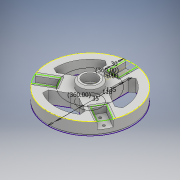
# Autodesk Inventor part: Base1
Saved by Autodesk Inventor 2017 (Build 210142000, 142)
## iProperties
Created: 2016-12-27
Part Number: Base1
Material: Generic
Document SubType Name: Modeling
Designer: Samanth
Density: 1 g/cm^3
Appearance: Default
Author: Samanth
Autodesk Inventor part; units mm, degrees
ref_plane "YZ Plane" through (0, 0, 0) normal (1, 0, 0) x (0, 1, 0)
ref_plane "XZ Plane" through (0, 0, 0) normal (0, 1, 0) x (-1, 0, 0)
ref_plane "XY Plane" through (0, 0, 0) normal (0, 0, 1) x (1, 0, 0)
sketch "Sketch1" plane through (0, 0, 0) normal (0, 0, 1) x (1, 0, 0)
  circle A0 centre (0, 0) radius 55
  circle A1 centre (0, 0) radius 17.5
  line L0 (-17.5, 0) -> (-17.5, 52.1416)
  line L1 (17.5, 0) -> (17.5, 52.1416)
  line L2 (8.75, -15.1554) -> (-36.406, -41.2263)
  line L3 (-8.75, 15.1554) -> (-53.906, -10.9154)
  circle A2 centre (0, 0) radius 17.5
  circle A3 centre (0, 0) radius 55
  line L4 (8.75, 15.1554) -> (53.906, -10.9154)
  line L5 (-8.75, -15.1554) -> (36.406, -41.2263)
  circle A4 centre (0, 0) radius 17.5
  circle A5 centre (0, 0) radius 55
  circle A6 centre (0, 0) radius 67.5
  line L6 (-36.406, -41.2263) -> (0, -20.2073)
  line L7 (36.406, -41.2263) -> (0, -20.2073)
  line L8 (53.906, -10.9154) -> (17.5, 10.1036)
  line L9 (17.5, 10.1036) -> (17.5, 52.1416)
  line L10 (-17.5, 10.1036) -> (-53.906, -10.9154)
  line L11 (-17.5, 52.1416) -> (-17.5, 10.1036)
  circle A7 centre (0, 0) radius 20.2073
  dimension "d0" = 110
  dimension "d1" = 35
  dimension "d4" = 360
  dimension "d6" = 135
  constraints: 24 end point, 12 point on circle, 8 coincident, 7 centre point, 6 point on line, 4 collinear, 2 tangent, 1 parallel, 1 vertical, 32 other
  measures "d0" diameter of A0
  measures "d1" diameter of A1
  measures "d6" diameter of A6
sketch "Sketch2" plane through (0, 0, 0) normal (0, 0, 1) x (1, 0, 0)
  circle A0 centre (0, 0) radius 67.5
  arc A1 (-17.5, 52.1416) -> (17.5, 52.1416) centre (0, 0) ccw
  line L0 (-17.5, 52.1416) -> (-17.5, 10.0984)
  line L1 (17.5, 10.0245) -> (17.5, 52.1416)
  line L2 (-36.406, -41.2263) -> (0, -20.2037)
  line L3 (-53.9044, -10.9232) -> (-17.5, 10.0984)
  arc A2 (-53.9044, -10.9232) -> (-36.406, -41.2263) centre (0, 0) ccw
  arc A3 (36.406, -41.2263) -> (53.906, -10.9154) centre (-0.0004, 0.0003) ccw
  arc A4 (-17.5, 52.1416) -> (17.5, 52.1416) centre (0, 0) ccw
  line L4 (36.406, -41.2263) -> (0, -20.2037)
  line L5 (-8.4334, -15.3339) -> (-9.065, -14.9691)
  line L6 (53.906, -10.9154) -> (17.5, 10.0245)
  arc A5 (-9.065, -14.9691) -> (-8.4334, -15.3339) centre (0, 0) ccw
  dimension "d7" = 135
  dimension "d8" = 110
  constraints: 14 end point, 13 point on circle, 6 centre point, 3 coincident, 2 parallel, 1 concentric
  measures "d7" diameter of A0
  measures "d8" diameter of A1
extrude "Extrusion1" add sketch "Sketch2" along normal blind 20 contours A0 | L6 L1 A1
sketch "Sketch3" plane through (0, 0, 20) normal (0, 0, 1) x (1, 0, 0)
  arc A0 (11.1455, 13.4917) -> (5.9543, 16.4559) centre (0, 0) ccw
  arc A1 (53.9044, -10.9232) -> (17.5, 52.1416) centre (0, 0) ccw
  line L0 (17.5, 9.8634) -> (17.5, 52.1416)
  arc A2 (53.9044, -10.9232) -> (17.5, 52.1416) centre (0, 0) ccw
  line L1 (53.9044, -10.9232) -> (17.5, 9.8634)
  dimension "d12" = 35
  constraints: 6 point on circle, 4 end point, 3 centre point, 2 coincident, 2 point on line, 2 tangent, 1 concentric, 1 vertical
  measures "d12" diameter of A0
extrude "Extrusion2" cut sketch "Sketch3" against normal blind 20
sketch "Sketch4" plane through (0, 0, 20) normal (0, 0, 1) x (1, 0, 0)
  circle A0 centre (0, 0) radius 7.4154
  constraints: 1 centre point, 1 coincident
extrude "Extrusion3" cut sketch "Sketch4" against normal blind 20
sketch "Sketch5" plane through (0, 0, 0) normal (0, 1, 0) x (-1, 0, 0)
  point P0 (0, 0)
sketch "Sketch6" plane through (0, 0, 20) normal (0, 0, 1) x (1, 0, 0)
  line L0 (0, 0) -> (0.0116, 67.4956) construction
  arc A0 (0, 67.5) -> (-9.3942, 66.8431) centre (0, 0) ccw
  line L1 (0, 0) -> (-9.3942, 66.8431) construction
  line L2 (0, 0) -> (0, 67.5) construction
  arc A1 (9.3942, 66.8431) -> (0, 67.5) centre (0, 0) ccw
  line L3 (0, 0) -> (9.3942, 66.8431) construction
  line L4 (0, 0) -> (0, 67.5) construction
  circle A2 centre (0, 0) radius 67.5 projected
  line L5 (-9.3942, 66.8431) -> (-9.3942, 36.8431)
  line L6 (-9.3942, 36.8431) -> (9.3942, 36.8431)
  line L7 (9.3942, 36.8431) -> (9.3942, 66.8431)
  line L8 (-27.21, -26.5571) -> (-36.6041, -10.2859)
  line L9 (-53.1907, -41.5571) -> (-27.21, -26.5571)
  line L10 (-36.6041, -10.2859) -> (-62.5849, -25.2859)
  arc A3 (-58.4567, -33.75) -> (-53.1907, -41.5571) centre (0, 0) ccw
  arc A4 (-62.5849, -25.2859) -> (-58.4567, -33.75) centre (0, 0) ccw
  line L11 (36.6041, -10.2859) -> (27.21, -26.5571)
  line L12 (62.5849, -25.2859) -> (36.6041, -10.2859)
  line L13 (27.21, -26.5571) -> (53.1907, -41.5571)
  arc A5 (58.4567, -33.75) -> (62.5849, -25.2859) centre (0, 0) ccw
  arc A6 (53.1907, -41.5571) -> (58.4567, -33.75) centre (0, 0) ccw
  dimension "d18" = 8
  dimension "d19" = 8
  dimension "d20" = 30
  dimension "d23" = 360
  constraints: 28 end point, 12 point on circle, 6 centre point, 5 coincident, 2 perpendicular, 1 point on line, 1 vertical, 42 other
  measures "d18" angle of L2 L1
  measures "d19" angle of L3 L4
  measures "d20" distance of L5.start L5.end
sketch "Sketch7" plane through (0, 0, 20) normal (0, 0, 1) x (1, 0, 0)
  circle A0 centre (0, 0) radius 67.5 projected
  line L0 (-9.3706, 66.8464) -> (-9.3706, 36.8464)
  line L1 (-9.3706, 36.8464) -> (9.4008, 36.8464)
  line L2 (9.4008, 36.8464) -> (9.4008, 66.8422)
  arc A1 (9.4008, 66.8422) -> (-9.3706, 66.8464) centre (0, 0) ccw
  line L3 (62.5849, -25.286) -> (36.6046, -10.2852)
  line L4 (36.6046, -10.2852) -> (27.1854, -26.5985)
  line L5 (27.1854, -26.5985) -> (53.1882, -41.5604)
  arc A2 (53.1882, -41.5604) -> (62.5849, -25.286) centre (0, 0) ccw
  arc A3 (-62.5682, -25.3273) -> (-53.1551, -41.6027) centre (0, 0) ccw
  line L6 (-62.5682, -25.3273) -> (-36.6095, -10.2891)
  line L7 (-36.6095, -10.2891) -> (-27.1612, -26.5985)
  line L8 (-53.1864, -41.5627) -> (-27.1612, -26.5985)
  dimension "d25" = 30
  dimension "d26" = 30
  dimension "d27" = 30
  constraints: 18 end point, 9 point on circle, 4 perpendicular, 3 centre point, 1 vertical, 10 other
  measures "d25" distance of L0.start L0.end
  measures "d26" distance of L3.start L3.end
  measures "d27" distance of L6.start L6.end
extrude "Extrusion4" cut sketch "Sketch7" against normal blind 12 contours L2 L1 L0 A0 | A0 L5 L4 L3 | L6 L7 L8 A0
sketch "Sketch8" plane through (0, 0, 8) normal (0, 0, 1) x (1, 0, 0)
  point P0 (0, 0)
sketch "Sketch9" plane through (0, 0, 8) normal (0, 0, 1) x (1, 0, 0)
  line L0 (9.4008, 36.8464) -> (-9.3706, 36.8464) projected
  line L1 (0.0151, 36.8464) -> (0.0151, 44.8464)
  line L2 (0.0151, 44.8464) -> (0.0151, 60.8464)
  circle A0 centre (0.0151, 44.8464) radius 2
  circle A1 centre (0.0151, 60.8464) radius 2
  circle A2 centre (-38.8457, -22.4101) radius 2
  circle A3 centre (-52.7021, -30.4101) radius 2
  circle A4 centre (38.8306, -22.4363) radius 2
  circle A5 centre (52.687, -30.4363) radius 2
  point P0 (0, 0)
  dimension "d30" = 8
  dimension "d31" = 16
  dimension "d32" = 4
  dimension "d33" = 4
  dimension "d36" = 360
  constraints: 6 centre point, 4 end point, 2 coincident, 1 midpoint, 1 point on line, 1 vertical, 13 other
  measures "d30" distance of L1.start L1.end
  measures "d31" distance of L1.end L2.end
  measures "d32" diameter of A0
  measures "d33" diameter of A1
extrude "Extrusion5" cut sketch "Sketch9" against normal blind 12
chamfer "Chamfer1" distance 2 angle 45 1 edges at (-67.5, 0, 0)
chamfer "Chamfer2" distance 8 angle 45 9 edges at (0, -20.2037, 10) (17.5, 52.1416, 10) (-17.5, 10.0984, 10) (17.5, 9.8634, 10) (36.406, -41.2263, 10) (-17.5, 52.1416, 10) (-53.9044, -10.9232, 10) (-36.406, -41.2263, 10) (53.9044, -10.9232, 10)
chamfer "Chamfer3" distance 3 angle 45 9 edges at (9.4008, 51.8443, 20) (0.0151, 36.8464, 20) (-9.3706, 51.8464, 20) (-49.5889, -17.8082, 20) (-31.8854, -18.4438, 20) (-40.1738, -34.0806, 20) (31.895, -18.4418, 20) (40.1868, -34.0794, 20) (49.5947, -17.7856, 20)
sketch "Sketch10" plane through (0, 0, 20) normal (0, 0, 1) x (1, 0, 0)
  circle A0 centre (0, 0) radius 11.5
  circle A1 centre (0, 0) radius 17.5124
  dimension "d49" = 23
  constraints: 2 centre point, 2 coincident
  measures "d49" diameter of A0
extrude "Extrusion6" add sketch "Sketch10" along normal blind 12
sketch "Sketch11" plane through (0, 0, 0) normal (0, 0, -1) x (-1, 0, 0)
  circle A0 centre (0, 0) radius 11.5
  dimension "d52" = 23
  constraints: 1 centre point, 1 coincident
  measures "d52" diameter of A0
extrude "Extrusion7" cut sketch "Sketch11" against normal blind 10
chamfer "Chamfer4" distance 3 angle 45 1 edges at (-17.5124, 0, 32)
body "Solid1"
